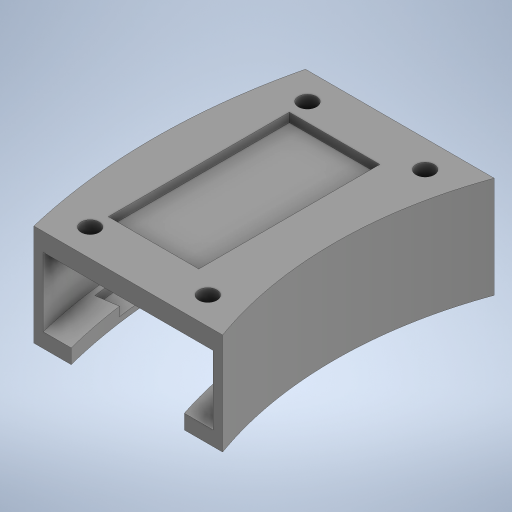
# Autodesk Inventor part: Battery Cage Second Iteration
Saved by Autodesk Inventor 2023 (Build 270158000, 158)
## iProperties
Created: 2023-02-13
Part Number: Battery Cage Second Iteration
Material: PLA 33 Plastic
Document SubType Name: Modeling
Designer: mihal
Density: 0.4135 g/cm^3
Appearance: Generic
Author: mihal
Autodesk Inventor part; units mm, degrees
ref_plane "YZ Plane" through (0, 0, 0) normal (1, 0, 0) x (0, 1, 0)
ref_plane "XZ Plane" through (0, 0, 0) normal (0, 1, 0) x (-1, 0, 0)
ref_plane "XY Plane" through (0, 0, 0) normal (0, 0, 1) x (1, 0, 0)
sketch "Sketch1" plane through (0, 0, 0) normal (0, 1, 0) x (-1, 0, 0)
  line L0 (0, 0) -> (140, 0)
  line L1 (140, 0) -> (140, -150)
  line L2 (140, -150) -> (0, -150)
  line L3 (0, -150) -> (0, 0)
  dimension "d0" = 140
  dimension "d1" = 150
  constraints: 8 end point, 2 parallel, 1 horizontal, 1 perpendicular
  measures "d0" distance of L1.end L2.end
  measures "d1" distance of L0.end L1.end
extrude "Extrusion1" add sketch "Sketch1" along normal blind 60
sketch "Sketch2" plane through (0, 0, 0) normal (0, -1, 0) x (1, 0, 0)
  line L0 (0, 0) -> (0, -150) projected
  line L1 (0, -75) -> (200, -75) construction
  circle A0 centre (200, -75) radius 215
  circle A1 centre (200, -75) radius 320
  circle A2 centre (200, -75) radius 330
  circle A3 centre (200, -75) radius 220
  circle A4 centre (200, -75) radius 365
  circle A5 centre (200, -75) radius 240
  circle A6 centre (200, -75) radius 300
  dimension "d4" = 200
  dimension "d5" = 430
  dimension "d7" = 10
  dimension "d8" = 5
  dimension "d9" = 100
  dimension "d10" = 730
  dimension "d13" = 60
  dimension "d14" = 20
  constraints: 7 centre point, 7 coincident, 2 end point, 1 horizontal, 1 midpoint
  measures "d4" distance of L1.start L1.end
  measures "d5" diameter of A0
  measures "d7" radial gap between concentric circles of A2 A1
  measures "d8" radial gap between concentric circles of A3 A0
  measures "d9" radial gap between concentric circles of A1 A3
  measures "d10" diameter of A4
  measures "d13" radial gap between concentric circles of A6 A5
  measures "d14" radial gap between concentric circles of A5 A3
extrude "Extrusion2" cut sketch "Sketch2" against normal blind 80 contours A0 | A2 | A3 | A4
extrude "Extrusion3" cut sketch "Sketch2" against normal blind 50 contours A6
sketch "Sketch3" plane through (0, 50, 0) normal (0, -1, 0) x (1, 0, 0)
  arc A0 (-90.4738, 0) -> (-90.4738, -150) centre (200, -75) ccw projected
  line L0 (-111.0868, 0) -> (-90.4738, 0) projected
  arc A1 (-111.0868, 0) -> (-111.0868, -150) centre (200, -75) ccw projected
  line L1 (-90.4738, -150) -> (-111.0868, -150) projected
  arc A2 (-27.9803, 0) -> (-27.9803, -150) centre (200, -75) ccw projected
  line L2 (-6.8212, -150) -> (-27.9803, -150) projected
  arc A3 (-6.8212, 0) -> (-6.8212, -150) centre (200, -75) ccw projected
  line L3 (-27.9803, 0) -> (-6.8212, 0) projected
  circle A4 centre (200, -75) radius 240
  circle A5 centre (200, -75) radius 300
  circle A6 centre (200, -75) radius 315
  circle A7 centre (200, -75) radius 225
  point P0 (-12.132, -150)
  point P1 (-12.132, 0)
  point P2 (-105.9412, 0)
  point P3 (-105.9412, -150)
  dimension "d47" = 480
  dimension "d48" = 15
  dimension "d49" = 15
  constraints: 4 coincident, 3 centre point, 3 other
  measures "d47" diameter of A4
  measures "d48" radial gap between concentric circles of A7 A4
extrude "Extrusion4" cut sketch "Sketch3" along normal blind 38 contours A0 L1 A6 L0 | L3 A7 L2 A2
sketch "Sketch4" plane through (0, 12, 0) normal (0, 1, 0) x (1, 0, 0)
  circle A0 centre (200, 75) radius 220 projected
  circle A1 centre (200, 75) radius 320 projected
  circle A2 centre (200, 75) radius 300 projected
  circle A3 centre (200, 75) radius 240 projected
  line L0 (200, 75) -> (-116.8858, 30.4646)
  arc A4 (-111.0868, 150) -> (-111.0868, 0) centre (200, 75) ccw projected
  arc A5 (-27.9803, 150) -> (-27.9803, 0) centre (200, 75) ccw projected
  line L1 (200, 75) -> (-116.8858, 119.5354)
  line L2 (-111.0868, 0) -> (-111.0868, 150) construction
  arc A6 (-121.3643, 150) -> (-121.3643, 0) centre (200, 75) ccw projected
  line L3 (-111.0868, 75) -> (200, 75) construction
  circle A7 centre (200, 75) radius 228
  circle A8 centre (200, 75) radius 312
  line L4 (-111.0868, 150) -> (-6.8212, 150)
  line L5 (-27.9803, 0) -> (-90.4738, 0) projected
  line L6 (-6.8212, 0) -> (-111.0868, 0)
  point P0 (0, 0)
  point P1 (-17.859, 105.6181)
  point P2 (-37.6643, 108.4015)
  point P3 (-37.6643, 41.5985)
  point P4 (-17.859, 44.3819)
  point P5 (-97.0804, 116.7519)
  point P6 (-116.8858, 30.4646)
  point P7 (-97.0804, 33.2481)
  point P8 (-25.7811, 43.2685)
  point P9 (-25.7811, 106.7315)
  point P10 (-108.9636, 118.422)
  point P11 (-108.9636, 31.578)
  point P12 (-1.4944, 0)
  point P13 (-15.3114, 150)
  point P14 (-15.3114, 0)
  point P15 (-102.8514, 0)
  point P16 (-102.8514, 150)
  dimension "d19" = 16
  dimension "d22" = 8
  dimension "d23" = 8
  constraints: 12 end point, 4 point on circle, 2 centre point, 2 coincident, 2 horizontal, 1 midpoint, 1 point on line, 2 other
  measures "d19" angle of L0 L1
  measures "d22" radial gap between concentric circles of A1 A8
  measures "d23" radial gap between concentric circles of A0 A7
extrude "Extrusion5" cut sketch "Sketch4" against normal blind 7 contours A7 L0 A3 L1 | A2 L0 A8 L1
extrude "Extrusion6" [suppressed]
sketch "Sketch5" plane through (0, 0, 0) normal (0, -1, 0) x (1, 0, 0)
  circle A0 centre (200, -75) radius 330 projected
  circle A1 centre (200, -75) radius 215 projected
  circle A2 centre (200, -75) radius 322
  circle A3 centre (200, -75) radius 223
  circle A4 centre (200, -75) radius 215
  circle A5 centre (200, -75) radius 330
  point P0 (0, 0)
  dimension "d26" = 8
  dimension "d27" = 8
  constraints: 4 centre point, 4 coincident, 2 concentric
  measures "d26" radial gap between concentric circles of A1 A3
  measures "d27" radial gap between concentric circles of A0 A2
extrude "Extrusion7" [suppressed]
sketch "Sketch6" plane through (0, 60, 0) normal (0, 1, 0) x (1, 0, 0)
  line L0 (-70, 75) -> (-45, 75)
  line L1 (-45, 75) -> (-45, 25)
  line L2 (-45, 25) -> (-70, 25)
  line L3 (-70, 25) -> (-70, 75)
  line L4 (-70, 75) -> (-95, 75)
  line L5 (-95, 75) -> (-95, 25)
  line L6 (-95, 25) -> (-70, 25)
  line L7 (-70, 25) -> (-70, 75)
  line L8 (-70, 75) -> (-95, 75)
  line L9 (-95, 75) -> (-95, 125)
  line L10 (-95, 125) -> (-70, 125)
  line L11 (-70, 125) -> (-70, 75)
  line L12 (-70, 75) -> (-45, 75)
  line L13 (-45, 75) -> (-45, 125)
  line L14 (-45, 125) -> (-70, 125)
  line L15 (-70, 125) -> (-70, 75)
  arc A0 (-111.0868, 150) -> (-111.0868, 0) centre (200, 75) ccw projected
  line L16 (-111.0868, 0) -> (-6.8212, 0) projected
  arc A1 (-6.8212, 150) -> (-6.8212, 0) centre (200, 75) ccw projected
  line L17 (-6.8212, 150) -> (-111.0868, 150) projected
  line L18 (-120, 75) -> (-20, 75) construction
  line L19 (-70, 75) -> (-70, 150) construction
  line L20 (-70, 75) -> (-70, 0) construction
  dimension "d37" = 25
  dimension "d38" = 50
  dimension "d39" = 25
  dimension "d40" = 50
  dimension "d41" = 25
  dimension "d42" = 50
  dimension "d43" = 25
  dimension "d44" = 50
  constraints: 38 end point, 8 parallel, 4 horizontal, 4 perpendicular, 3 point on line, 2 point on circle, 1 midpoint, 1 vertical
  measures "d37" distance of L1.end L2.end
  measures "d38" distance of L0.end L1.end
  measures "d39" distance of L6.end L5.end
  measures "d40" distance of L5.end L4.end
  measures "d41" distance of L9.end L10.end
  measures "d42" distance of L8.end L9.end
  measures "d43" distance of L14.end L13.end
  measures "d44" distance of L13.end L12.end
extrude "Extrusion8" cut sketch "Sketch6" against normal blind 5 contours L11 L14 L13 L0 | L0 L1 L2 L3 | L3 L6 L5 L4 | L4 L9 L10 L11
sketch "Sketch7" plane through (0, 60, 0) normal (0, -1, 0) x (1, 0, 0)
  line L0 (-12.132, -150) -> (-105.9412, -150) projected
  arc A0 (-12.132, 0) -> (-12.132, -150) centre (200, -75) ccw projected
  line L1 (-105.9412, 0) -> (-12.132, 0) projected
  arc A1 (-105.9412, 0) -> (-105.9412, -150) centre (200, -75) ccw projected
  circle A2 centre (200, -75) radius 227.5
  line L2 (0, 0) -> (200, 0)
  circle A3 centre (200, -75) radius 312.5
  line L3 (-45, -125) -> (-45, -25) projected
  line L4 (-95, -125) -> (-45, -125) projected
  line L5 (-95, -25) -> (-95, -125) projected
  line L6 (-45, -25) -> (-95, -25) projected
  line L7 (-95, -25) -> (-95, -15) construction
  line L8 (-95, -25) -> (-85, -25) construction
  line L9 (-45, -25) -> (-45, -15) construction
  circle A4 centre (-95, -15) radius 5
  line L10 (-95, -125) -> (-95, -135) construction
  line L11 (-95, -125) -> (-85, -125) construction
  line L12 (-45, -15) -> (-30, -15) construction
  circle A5 centre (-30, -15) radius 5
  line L13 (-45, -125) -> (-45, -135) construction
  line L14 (-45, -135) -> (-30, -135) construction
  circle A6 centre (-95, -135) radius 5
  circle A7 centre (-30, -135) radius 5
  dimension "d50" = 455
  dimension "d52" = 625
  dimension "d53" = 10
  dimension "d54" = 90
  dimension "d55" = 10
  dimension "d56" = 10
  dimension "d57" = 90
  dimension "d59" = 15
  dimension "d60" = 10
  dimension "d61" = 10
  dimension "d62" = 10
  constraints: 18 end point, 6 centre point, 6 coincident, 4 horizontal, 4 vertical, 3 perpendicular
  measures "d50" diameter of A2
  measures "d52" diameter of A3
  measures "d53" distance of L5.start L7.end
  measures "d54" angle of L8 L7
  measures "d55" diameter of A4
  measures "d56" distance of L4.start L10.end
  measures "d57" angle of L10 L11
  measures "d59" distance of L9.end L12.end
  measures "d60" diameter of A5
  measures "d61" diameter of A6
  measures "d62" diameter of A7
extrude "Extrusion9" cut sketch "Sketch7" along normal blind 10 contours A4 | A5 | A6 | A7
sketch "Sketch8" plane through (0, 0, 0) normal (0, -1, 0) x (1, 0, 0)
  arc A0 (-90.4738, 0) -> (-90.4738, -150) centre (200, -75) ccw projected
  line L0 (-111.0868, 0) -> (-90.4738, 0) projected
  arc A1 (-111.0868, 0) -> (-111.0868, -150) centre (200, -75) ccw projected
  line L1 (-90.4738, -150) -> (-111.0868, -150) projected
  arc A2 (-27.9803, 0) -> (-27.9803, -150) centre (200, -75) ccw projected
  line L2 (-6.8212, -150) -> (-27.9803, -150) projected
  arc A3 (-6.8212, 0) -> (-6.8212, -150) centre (200, -75) ccw projected
  line L3 (-27.9803, 0) -> (-6.8212, 0) projected
  point P0 (0, 0)
extrude "Extrusion10" cut sketch "Sketch8" against normal blind 4
sketch "Sketch9" plane through (0, 5, 0) normal (0, 1, 0) x (1, 0, 0)
  line L0 (-37.6643, 108.4015) -> (-25.7811, 106.7315) projected
  arc A0 (-37.6643, 108.4015) -> (-37.6643, 41.5985) centre (200, 75) ccw projected
  line L1 (-25.7811, 43.2685) -> (-37.6643, 41.5985) projected
  arc A1 (-25.7811, 106.7315) -> (-25.7811, 43.2685) centre (200, 75) ccw projected
  line L2 (-97.0804, 33.2481) -> (-108.9636, 31.578) projected
  arc A2 (-97.0804, 116.7519) -> (-97.0804, 33.2481) centre (200, 75) ccw projected
  line L3 (-108.9636, 118.422) -> (-97.0804, 116.7519) projected
  arc A3 (-108.9636, 118.422) -> (-108.9636, 31.578) centre (200, 75) ccw projected
  point P0 (0, 0)
extrude "Extrusion11" add sketch "Sketch9" along normal blind 2
body "Solid1"
